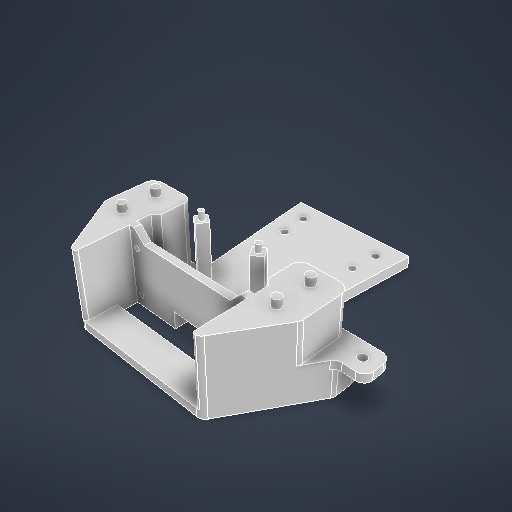
# Autodesk Inventor part: Front Bridge
Saved by Autodesk Inventor 2025 (Build 290162000, 162)
## iProperties
Created: 2024-05-23
Part Number: Front Bridge
Material: Generic
Document SubType Name: Modeling
Designer: DELL
Density: 1 g/cm^3
Appearance: Default
Mass: 43.2187 g
Surface Area: 102.411 cm^2
Volume: 43.2187 cm^3
Author: DELL
Autodesk Inventor part; units mm, degrees
ref_plane "YZ Plane" through (0, 0, 0) normal (1, 0, 0) x (0, 1, 0)
ref_plane "XZ Plane" through (0, 0, 0) normal (0, 1, 0) x (-1, 0, 0)
ref_plane "XY Plane" through (0, 0, 0) normal (0, 0, 1) x (1, 0, 0)
derived "Car_Plan.ipt"
sketch "Car_Sketch" plane through (0, 0, 0) normal (0, 1, 0) x (-1, 0, 0)
  line L0 (0, 0) -> (94, 0)
  line L1 (0, 0) -> (0, 105)
  line L2 (94, 0) -> (94, 105)
  line L3 (0, 105) -> (20, 105)
  line L4 (20, 105) -> (20, 190)
  line L5 (20, 190) -> (74, 190)
  line L6 (74, 190) -> (74, 105)
  line L7 (74, 105) -> (94, 105)
  line L8 (-5, 68) -> (-5, 0)
  line L9 (-5, 0) -> (-32, 0)
  line L10 (-32, 0) -> (-32, 68)
  line L11 (-32, 68) -> (-5, 68)
  line L12 (47, 190) -> (47, 0) construction
  line L13 (126, 68) -> (99, 68)
  line L14 (99, 68) -> (99, 0)
  line L15 (126, 0) -> (126, 68)
  line L16 (99, 0) -> (126, 0)
  line L17 (-5, 34) -> (99, 34) construction
  line L18 (0, 95) -> (94, 95) construction
  line L19 (-5, 190) -> (-32, 190)
  line L20 (-32, 122) -> (-5, 122)
  line L21 (-32, 190) -> (-32, 122)
  line L22 (-5, 122) -> (-5, 190)
  line L23 (-5, 156) -> (99, 156) construction
  line L24 (126, 122) -> (99, 122)
  line L25 (126, 190) -> (126, 122)
  line L26 (99, 190) -> (126, 190)
  line L27 (99, 122) -> (99, 190)
  line L28 (0, 156) -> (47, 34) construction
  line L29 (94, 156) -> (47, 34) construction
  line L30 (0, 156) -> (-174.2341, 34) construction
  line L31 (-5, 34) -> (-174.2341, 34) construction
  line L32 (8.9873, 132.6713) -> (47, 142.55) construction
  line L33 (85.0127, 132.6713) -> (47, 142.55) construction
sketch "Front_Bridge_Base" plane through (0, 0, 0) normal (0, 1, 0) x (-1, 0, 0)
  circle A0 centre (0, 156) radius 1.5
  circle A1 centre (94, 156) radius 1.5
  line L0 (-5, 161) -> (-5, 151)
  line L1 (-5, 151) -> (29.5, 151)
  line L2 (99, 151) -> (99, 161)
  line L3 (99, 161) -> (90, 161)
  line L4 (4, 161) -> (22, 190)
  line L5 (22, 190) -> (72, 190)
  line L6 (72, 190) -> (90, 161)
  line L7 (0, 156) -> (94, 156) construction
  line L8 (4, 161) -> (-5, 161)
  line L9 (40.95, 172.3) -> (53.05, 172.3)
  line L10 (53.05, 172.3) -> (53.05, 149.9)
  line L11 (53.05, 149.9) -> (40.95, 149.9)
  line L12 (40.95, 149.9) -> (40.95, 172.3)
  line L13 (47, 156) -> (47, 149.9) construction
  line L14 (32, 151) -> (37, 144)
  line L15 (37, 144) -> (57, 144)
  line L16 (57, 144) -> (62, 151)
  line L17 (47, 156) -> (47, 144) construction
  line L18 (32, 151) -> (62, 151)
  line L19 (62, 151) -> (64.5, 151)
  line L20 (29.5, 151) -> (24.5, 102)
  line L21 (24.5, 102) -> (69.5, 102)
  line L22 (69.5, 102) -> (64.5, 151)
  line L23 (64.5, 151) -> (99, 151)
  line L24 (29.5, 151) -> (32, 151)
  line L25 (4, 161) -> (4, 151)
  line L26 (90, 161) -> (90, 151)
  circle A2 centre (32, 109) radius 1.5
  circle A3 centre (33, 119) radius 1.5
  line L27 (47, 156) -> (47, 102) construction
  circle A4 centre (62, 109) radius 1.5
  circle A5 centre (61, 119) radius 1.5
  line L28 (9, 169.0556) -> (9, 151)
  line L29 (84.8333, 151) -> (84.5992, 150.8961)
  line L30 (85, 169.0556) -> (85, 151)
  line L31 (26, 190) -> (26, 151)
  line L32 (68, 190) -> (68, 151)
  circle A6 centre (17, 157) radius 1.5
  circle A7 centre (17, 169) radius 1.5
  circle A8 centre (77, 157) radius 1.5
  circle A9 centre (77, 169) radius 1.5
  line L33 (37.95, 162.3) -> (33.95, 162.3)
  line L34 (33.95, 162.3) -> (33.95, 172.3)
  line L35 (33.95, 172.3) -> (37.95, 172.3)
  line L36 (37.95, 172.3) -> (37.95, 162.3)
  circle A10 centre (47, 156) radius 17.5
  line L37 (47, 156) -> (61.3352, 145.9624) construction
  line L38 (47, 156) -> (32.6648, 145.9624) construction
  line L39 (38.6848, 155.6711) -> (35.4082, 153.3768)
  line L40 (35.4082, 153.3768) -> (33.1139, 156.6535)
  line L41 (38.6848, 155.6711) -> (36.3905, 158.9478)
  line L42 (36.3905, 158.9478) -> (33.1139, 156.6535)
  line L43 (55.3152, 155.6711) -> (58.5918, 153.3768)
  line L44 (58.5918, 153.3768) -> (60.8861, 156.6535)
  line L45 (60.8861, 156.6535) -> (57.6095, 158.9478)
  line L46 (57.6095, 158.9478) -> (55.3152, 155.6711)
  line L47 (59.2478, 157.8006) -> (56.9535, 154.524) construction
  circle A11 centre (58.1006, 156.1623) radius 1
  line L48 (37.0465, 154.524) -> (34.7522, 157.8006) construction
  circle A12 centre (35.8994, 156.1623) radius 1
  dimension "d130" = 3
  dimension "d131" = 3
  dimension "d132" = 5
  dimension "d134" = 5
  dimension "d136" = 5
  dimension "d137" = 5
  dimension "d138" = 4
  dimension "d139" = 5
  dimension "d140" = 34
  dimension "d143" = 50
  dimension "d168" = 16.3
  dimension "d169" = 12.1
  dimension "d170" = 22.4
  dimension "d173" = 6.05
  dimension "d174" = 12
  dimension "d175" = 20
  dimension "d176" = 15
  dimension "d214" = 45
  dimension "d215" = 54
  dimension "d216" = 35
  dimension "d221" = 3
  dimension "d222" = 3
  dimension "d223" = 32
  dimension "d224" = 42
  dimension "d225" = 14
  dimension "d226" = 15
  dimension "d252" = 5
  dimension "d253" = 5
  dimension "d254" = 4
  dimension "d255" = 4
  dimension "d277" = 3
  dimension "d281" = 3
  dimension "d282" = 3
  dimension "d283" = 3
  dimension "d284" = 8
  dimension "d285" = 8
  dimension "d286" = 8
  dimension "d287" = 8
  dimension "d288" = 6
  dimension "d289" = 18
  dimension "d290" = 6
  dimension "d291" = 18
  dimension "d353" = 4
  dimension "d354" = 10
  dimension "d355" = 3
  dimension "d367" = 35
  dimension "d368" = 35
  dimension "d369" = 35
  dimension "d373" = 4
  dimension "d375" = 4
  dimension "d378" = 4.5
  dimension "d379" = 7
  dimension "d381" = 4
  dimension "d382" = 4
  dimension "d383" = 7
  dimension "d384" = 4.5
  dimension "d386" = 2
  dimension "d387" = 2
  constraints: 98 end point, 28 perpendicular, 15 parallel, 13 centre point, 12 point on line, 10 midpoint, 5 equal length, 3 coincident, 2 point on circle, 2 symmetric about line, 1 collinear, 2 other
  measures "d130" diameter of A0
  measures "d131" diameter of A1
  measures "d132" distance from line of L0 L7.start
  measures "d134" distance from line of L1 point (0, 156)
  measures "d136" distance from line of L2 point (94, 156)
  measures "d137" distance from line of L3 point (94, 156)
  measures "d138" horizontal distance of L4.start point (0, 156)
  measures "d139" distance from line of L8 L7.start
  measures "d140" distance between parallel lines of L7 L5
  measures "d143" distance of L4.end L5.end
  measures "d168" distance from line of L9 L13.start
  measures "d169" distance of L10.end L11.end
  measures "d170" distance of L10.end L9.end
  measures "d173" distance between parallel lines of L12 L13
  measures "d174" distance of L17.end L13.start
  measures "d175" distance of L15.end L14.end
  measures "d176" distance from line of L17 L14.start
  measures "d214" distance of L20.end L21.end
  measures "d215" distance between parallel lines of L21 L7
  measures "d216" distance of L1.end L19.end
  measures "d221" diameter of A2
  measures "d222" diameter of A3
  measures "d223" distance from line of A3.centre L18
  measures "d224" distance from line of A2.centre L24
  measures "d225" distance from line of L27 A3.centre
  measures "d226" distance from line of L27 A2.centre
  measures "d252" distance between parallel lines of L28 L25
  measures "d253" distance between parallel lines of L26 L30
  measures "d254" distance from line of L4.end L31
  measures "d255" distance from line of L32 L5.end
  measures "d277" diameter of A6
  measures "d281" diameter of A7
  measures "d282" diameter of A8
  measures "d283" diameter of A9
  measures "d284" distance from line of L28 A6.centre
  measures "d285" distance from line of A7.centre L28
  measures "d286" distance from line of L30 A8.centre
  measures "d287" distance from line of L30 A9.centre
  measures "d288" distance from line of L1 A6.centre
  measures "d289" distance from line of L1 A7.centre
  measures "d290" distance from line of L23 A8.centre
  measures "d291" distance from line of L23 A9.centre
  measures "d353" distance of L34.end L35.end
  measures "d354" distance of L33.end L34.end
  measures "d355" distance between parallel lines of L36 L12
  measures "d367" diameter of A10
  measures "d368" angle of L7 L37
  measures "d369" angle of L7 L38
  measures "d373" distance of L39.start L39.end
  measures "d375" distance between parallel lines of L42 L39
  measures "d378" distance between parallel lines of L38 L39
  measures "d379" distance from line of L41 L37.start
  measures "d381" distance between parallel lines of L44 L46
  measures "d382" distance between parallel lines of L45 L43
  measures "d383" distance from line of L13.start L46
  measures "d384" distance between parallel lines of L37 L43
  measures "d386" diameter of A11
  measures "d387" diameter of A12
extrude "Base_1_Extrusion" add sketch "Front_Bridge_Base" along normal blind 3 contours L8 L25 L1 L0 | L4 L28 L1 L25 | L4 L5 L31 L1 L28 | L31 L5 L32 L23 L19 A10 L36 L35 L34 L24 L1 | L5 L6 L30 L23 L32 | A10 L34 L33 L36 L19 L18 L10 L9 L12 L24 | A10 L36 L33 L34 | L34 L35 L36 A10 | L6 L26 L23 L30 | L12 L9 L10 L18 | L3 L2 L23 L26 | A6 | A7 | A8 | A9 | L39 L40 L42 L41 | L46 L45 L44 L43 | A11 | A12
sketch "Base_2" plane through (0, 3, 0) normal (0, 1, 0) x (1, 0, 0)
  line L0 (-9, -169.0556) -> (-9, -151) projected
  line L1 (-4, -161) -> (-22, -190) projected
  line L2 (5, -151) -> (-29.5, -151) projected
  line L3 (-26, -190) -> (-26, -151) projected
  line L4 (-22, -190) -> (-72, -190) projected
  line L5 (-68, -190) -> (-68, -151) projected
  line L6 (-72, -190) -> (-90, -161) projected
  line L7 (-85, -169.0556) -> (-85, -151) projected
  line L8 (-64.5, -151) -> (-99, -151) projected
  point P0 (0, 0)
extrude "Base_2_Extrusion" add sketch "Base_2" along normal blind 14
extrude "Bottom_Base_Extrusion" add sketch "Front_Bridge_Base" against normal blind 10 contours L4 L28 L1 L25 | L4 L5 L31 L1 L28 | L31 L5 L32 L23 L19 A10 L36 L35 L34 L24 L1 | L5 L6 L30 L23 L32 | A10 L34 L33 L36 L19 L18 L10 L9 L12 L24 | A10 L36 L33 L34 | L34 L35 L36 A10 | L6 L26 L23 L30 | L12 L9 L10 L18 | A6 | A7 | A8 | A9 | L39 L40 L42 L41 | L46 L45 L44 L43 | A11 | A12
chamfer "Chamfer_For_Wheel_Anchor" distance 3 angle 28 2 edges at (-9, 10, 151) (-85, 10, 151) measured on face at (-84.5, 10, 151) measured on face at (-9.5, 10, 151)
sketch "Chassis_Connector" plane through (0, -10, 0) normal (0, -1, 0) x (1, 0, 0)
  line L0 (-29.5, 151) -> (-24.5, 102) projected
  line L1 (-24.5, 102) -> (-69.5, 102) projected
  line L2 (-69.5, 102) -> (-64.5, 151) projected
  line L3 (-29.5, 151) -> (-32, 151) projected
  line L4 (-32, 151) -> (-62, 151) projected
  line L5 (-62, 151) -> (-64.5, 151) projected
  circle A0 centre (-33, 119) radius 1.5 projected
  circle A1 centre (-32, 109) radius 1.5 projected
  circle A2 centre (-62, 109) radius 1.5 projected
  circle A3 centre (-61, 119) radius 1.5 projected
  point P0 (0, 0)
extrude "Chassis_Connector_Extrusion" add sketch "Chassis_Connector" against normal blind 4
extrude "Extrusion31" add sketch "Front_Bridge_Base" along normal blind 17 contours L39 L40 L42 L41 | L46 L45 L44 L43 | A11 | A12
extrude "Extrusion32" add sketch "Front_Bridge_Base" along normal blind 20 contours A11 | A12
sketch "Alignment_Pin" plane through (0, 17, 0) normal (0, 1, 0) x (1, 0, 0)
  circle A0 centre (-17, -157) radius 1.5 projected
  circle A1 centre (-17, -169) radius 1.5 projected
  circle A2 centre (-77, -169) radius 1.5 projected
  circle A3 centre (-77, -157) radius 1.5 projected
  point P0 (0, 0)
extrude "Alignment_Pin_Extrusion" add sketch "Alignment_Pin" along normal blind 3
move faces "Move1" translate (0, -9, 0) faces at (-43.4635, 3, 179.6493)
sketch "Ultrasonic_Sketch" plane through (-69.5, -6, 102) normal (0, 1, 0) x (1, 0, 0)
  line L0 (1.5, -88) -> (43.5, -88) projected
  line L1 (1.5, -49) -> (1.5, -88) construction
  line L2 (43.5, -88) -> (43.5, -49) construction
  line L3 (-0.5, -70) -> (45.5, -70)
  line L4 (45.5, -70) -> (45.5, -77)
  line L5 (45.5, -77) -> (-0.5, -77)
  line L6 (-0.5, -77) -> (-0.5, -70)
  line L7 (22.5, -77) -> (22.5, -88) construction
  line L8 (1.5, -88) -> (1.5, -49) construction
  line L9 (-0.5, -70) -> (-0.5, -67.5)
  line L10 (-0.5, -67.5) -> (45.5, -67.5)
  line L11 (45.5, -67.5) -> (45.5, -70)
  line L12 (-0.5, -67.5) -> (-0.5, -62.5)
  line L13 (45.5, -67.5) -> (45.5, -62.5)
  line L14 (45.5, -62.5) -> (43.5, -62.5)
  line L15 (43.5, -62.5) -> (43.5, -67.5)
  line L16 (-0.5, -62.5) -> (1.5, -62.5)
  line L17 (1.5, -62.5) -> (1.5, -67.5)
  point P0 (1.5, -77)
  point P1 (43.5, -77)
  point P2 (43.5, -70)
  point P3 (1.5, -70)
  point P4 (1.5, -77)
  point P5 (1.5, -70)
  point P6 (44.5, -62.5)
  dimension "d305" = 46
  dimension "d306" = 7
  dimension "d307" = 11
  dimension "d325" = 2.5
  dimension "d356" = 5
  dimension "d357" = 5
  constraints: 28 end point, 9 perpendicular, 4 point on line, 3 midpoint, 3 parallel, 2 collinear
  measures "d305" distance of L4.end L5.end
  measures "d306" distance of L4.end L3.end
  measures "d307" distance between parallel lines of L0 L5
  measures "d325" distance between parallel lines of L3 L10
  measures "d356" distance from line of point (44.5, -62.5) L10
  measures "d357" distance between parallel lines of L16 L10
extrude "Ultrasonic_Hole_Extrusion" cut sketch "Ultrasonic_Sketch" along normal through all both and the other way through all contours L3 L4 L5 L6
move faces "Move4" translate (-2, 0, 0) faces at (-68, 1.6667, 186.3333)
move faces "Move5" translate (2, 0, 0) faces at (-26, 9.3333, 182.6667)
move faces "Move6" translate (0, -1, 0) faces at (-39.3333, -6, 182.6667)
extrude "Ultrasonic_Holder_Extrusion" add sketch "Ultrasonic_Sketch" along normal blind 19 contours L9 L10 L11 L3
sketch "Ultrasonic_Holder_Sketch" plane through (-70, -10, 172) normal (0, 0, 1) x (1, 0, 0)
  circle A0 centre (2.35, 20.15) radius 1
  circle A1 centre (43.65, 20.15) radius 1
  circle A2 centre (2.35, 3.85) radius 1
  circle A3 centre (43.65, 3.85) radius 1
  line L0 (0.5, 22) -> (45.5, 22)
  line L1 (45.5, 22) -> (45.5, 2)
  line L2 (45.5, 2) -> (0.5, 2)
  line L3 (0.5, 2) -> (0.5, 22)
  line L4 (0, 0) -> (46, 0) projected
  line L5 (23, 2) -> (23, 0) construction
  line L6 (46, 0) -> (0, 0) projected
  line L7 (17, 0) -> (17, 6)
  line L8 (17, 6) -> (29, 6)
  line L9 (29, 6) -> (29, 0)
  line L10 (23, 6) -> (23, 0) construction
  point P0 (70, 10)
  point P1 (17, 0)
  point P2 (29, 0)
  dimension "d326" = 2
  dimension "d327" = 2
  dimension "d328" = 2
  dimension "d329" = 2
  dimension "d330" = 20
  dimension "d331" = 2
  dimension "d332" = 45
  dimension "d333" = 1.85
  dimension "d334" = 1.85
  dimension "d335" = 1.85
  dimension "d336" = 1.85
  dimension "d337" = 1.85
  dimension "d338" = 1.85
  dimension "d339" = 1.85
  dimension "d340" = 1.85
  dimension "d349" = 12
  dimension "d350" = 6
  constraints: 18 end point, 8 perpendicular, 4 centre point, 3 midpoint, 2 point on line
  measures "d326" diameter of A0
  measures "d327" diameter of A1
  measures "d328" diameter of A2
  measures "d329" diameter of A3
  measures "d330" distance of L2.end L0.start
  measures "d331" distance between parallel lines of L2 L4
  measures "d332" distance between parallel lines of L1 L3
  measures "d333" distance from line of L0 A0.centre
  measures "d334" distance from line of L3 A0.centre
  measures "d335" distance from line of L0 A1.centre
  measures "d336" distance from line of L1 A1.centre
  measures "d337" distance from line of L3 A2.centre
  measures "d338" distance from line of L2 A2.centre
  measures "d339" distance from line of L1 A3.centre
  measures "d340" distance from line of L2 A3.centre
  measures "d349" distance of L8.end L7.end
  measures "d350" distance of L7.start L7.end
extrude "Ultrasonic_Screw_Hole_Extrusion" cut sketch "Ultrasonic_Sketch" along normal up to surface (23 mm away) contours L12 L16 L17 L10 | L10 L15 L14 L13
extrude "Ultrasonic_Holder_Hole_Extrusion" cut sketch "Ultrasonic_Holder_Sketch" against normal up to surface (2.5 mm away) contours A0 | A1 | A2 | A3
extrude "Ultrasonic_Holder_Hole_2_Extrusion" cut sketch "Ultrasonic_Holder_Sketch" against normal blind 10 contours L7 L8 L9 L2 | L2 L9 L4 L7
chamfer "Chamfer8" distance 4 angle 45 2 edges at (-68, 13, 170.75) (-26, 13, 170.75)
chamfer "Chamfer7" distance 2 angle 45 2 edges at (-26, 5.5, 164.5) (-68, 5.5, 164.5)
fillet "Fillet14" radius 3 16 edges at (-22, 3.5, 190) (-72, 3.5, 190) (-9, 10, 169.0556) (-4, -5, 161) (-4, -5, 151) (-9, 10, 152.5951) (-26, 5.5, 151) (-68, 5.5, 151) (-85, 10, 152.5951) (-85, 10, 169.0556) (-90, -5, 161) (-90, -5, 151) (-99, 1.5, 161) (-99, 1.5, 151) (5, 1.5, 161) (5, 1.5, 151)
fillet "Fillet15" radius 1 2 edges at (-70, 5, 190) (-24, 5, 190)
fillet "Fillet16" radius 3 2 edges at (-4.1245, 1.5, 161) (-89.8755, 1.5, 161)
body "Solid3"
